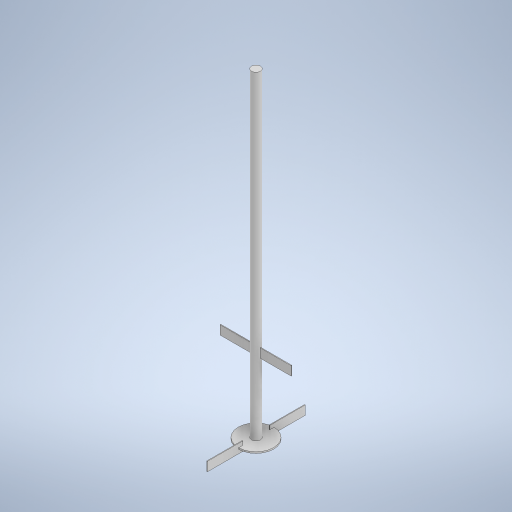
# Autodesk Inventor part: Mixer_1
Saved by Autodesk Inventor 2024 (Build 280153000, 153)
## iProperties
Created: 2024-10-31
Part Number: Mixer_1
Material: Generic
Document SubType Name: Modeling
Designer: raule
Density: 1 g/cm^3
Appearance: Default
Author: raule
Autodesk Inventor part; units mm, degrees
ref_plane "YZ Plane" through (0, 0, 0) normal (1, 0, 0) x (0, 1, 0)
ref_plane "XZ Plane" through (0, 0, 0) normal (0, 1, 0) x (-1, 0, 0)
ref_plane "XY Plane" through (0, 0, 0) normal (0, 0, 1) x (1, 0, 0)
sketch "Sketch1" plane through (0, 0, 0) normal (0, 1, 0) x (-1, 0, 0)
  circle A0 centre (0, 0) radius 12.7
  dimension "d0" = 25.4
  constraints: 1 centre point, 1 coincident
  measures "d0" diameter of A0
extrude "Extrusion1" add sketch "Sketch1" along normal blind 900
sketch "Sketch2" plane through (0, 0, 0) normal (0, -1, 0) x (1, 0, 0)
  circle A0 centre (0, 0) radius 50
  dimension "d3" = 100
  constraints: 1 centre point, 1 coincident
  measures "d3" diameter of A0
extrude "Extrusion2" add sketch "Sketch2" along normal blind 4
sketch "Sketch3" plane through (0, 0, 0) normal (1, 0, 0) x (0, 1, 0)
  line L0 (0, 50) -> (0, -50) projected
  line L1 (-4, 50) -> (-4, -50) projected
  line L2 (-14.7, -37.7) -> (10.7, -37.7)
  line L3 (10.7, -37.7) -> (10.7, -137.7)
  line L4 (10.7, -137.7) -> (-14.7, -137.7)
  line L5 (-14.7, -137.7) -> (-14.7, -37.7)
  line L6 (0, -12.7) -> (900, -12.7) projected
  line L7 (0, 12.7) -> (900, 12.7) projected
  line L8 (0, 0) -> (76.0488, 0) construction
  line L9 (-14.7, 37.7) -> (10.7, 37.7)
  line L10 (10.7, 37.7) -> (10.7, 137.7)
  line L11 (10.7, 137.7) -> (-14.7, 137.7)
  line L12 (-14.7, 137.7) -> (-14.7, 37.7)
  dimension "d6" = 100
  dimension "d7" = 25
  dimension "d8" = 25.4
  dimension "d9" = 10.7
  constraints: 18 end point, 4 symmetric about line, 2 horizontal, 2 parallel, 1 perpendicular
  measures "d6" distance of L2.end L3.end
  measures "d7" distance between parallel lines of L6 L2
  measures "d8" distance of L3.end L4.end
  measures "d9" distance between parallel lines of L1 L5
extrude "Extrusion3" add sketch "Sketch3" along normal mid plane 2 contours L9 L12 L11 L10 | L2 L3 L4 L5
sketch "Sketch4" plane through (0, 0, 0) normal (0, 0, 1) x (1, 0, 0)
  line L0 (-100, 225.4) -> (100, 225.4)
  line L1 (100, 225.4) -> (100, 200)
  line L2 (100, 200) -> (-100, 200)
  line L3 (-100, 200) -> (-100, 225.4)
  line L4 (-12.7, 0) -> (-12.7, 900) projected
  line L5 (12.7, 0) -> (12.7, 900) projected
  line L6 (1, 0) -> (50, 0) projected
  point P0 (0, 0)
  point P1 (12.7, 225.4)
  point P2 (12.7, 200)
  point P3 (-12.7, 200)
  point P4 (-12.7, 225.4)
  dimension "d12" = 25.4
  dimension "d13" = 200
  dimension "d14" = 87.3
  dimension "d15" = 87.3
  dimension "d16" = 200
  constraints: 8 end point, 2 parallel, 1 horizontal, 1 perpendicular
  measures "d12" distance of L2.end L0.start
  measures "d13" distance of L0.start L0.end
  measures "d14" distance between parallel lines of L4 L3
  measures "d15" distance between parallel lines of L5 L1
  measures "d16" distance between parallel lines of L6 L2
extrude "Extrusion4" add sketch "Sketch4" along normal mid plane 2 contours L0 L4 L2 L3 | L0 L1 L2 L5
body "Solid1"
